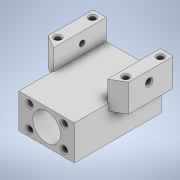
# Autodesk Inventor part: Губка-2
Saved by Autodesk Inventor 2022 (Build 260153000, 153)
## iProperties
Created: 2021-12-03
Part Number: Губка-2
Material: Типовые
Document SubType Name: Modeling
Designer: Украинцев
Density: 1 g/cm^3
Appearance: По умолчанию
Author: Украинцев
Autodesk Inventor part; units mm, degrees
ref_plane "YZ Plane" through (0, 0, 0) normal (1, 0, 0) x (0, 1, 0)
ref_plane "XZ Plane" through (0, 0, 0) normal (0, 1, 0) x (-1, 0, 0)
ref_plane "XY Plane" through (0, 0, 0) normal (0, 0, 1) x (1, 0, 0)
sketch "Эскиз1" plane through (0, 0, 0) normal (0, 1, 0) x (-1, 0, 0)
  line L0 (-40, 62.5) -> (40, 62.5)
  line L1 (40, 62.5) -> (40, -62.5)
  line L2 (40, -62.5) -> (-40, -62.5)
  line L3 (-40, -62.5) -> (-40, 62.5)
  line L4 (-40, 62.5) -> (40, -62.5) construction
  line L5 (40, 62.5) -> (-40, -62.5) construction
  line L6 (0, -62.5) -> (-58, -62.5)
  line L7 (-58, -62.5) -> (-58, 2.5)
  line L8 (-58, 2.5) -> (-39, 13.4697)
  line L9 (-58, -62.5) -> (-39, -62.5)
  line L10 (-39, -62.5) -> (-39, 13.4697)
  line L11 (0, 62.5) -> (0, -62.5)
  line L12 (0, -62.5) -> (58, -62.5)
  line L13 (58, -62.5) -> (58, 2.5)
  line L14 (58, 2.5) -> (39, 13.4697)
  line L15 (39, -62.5) -> (39, 13.4697)
  point P0 (0, 0)
  point P1 (-40, 12.8923)
  point P2 (40, 12.8923)
  dimension "d0" = 80
  dimension "d1" = 125
  dimension "d2" = 58
  dimension "d3" = 65
  dimension "d4" = 120
  dimension "d5" = 19
  constraints: 32 end point, 4 midpoint, 4 symmetric about line, 3 perpendicular, 2 horizontal, 2 parallel, 2 point on line, 1 vertical
  measures "d0" distance of L1.end L2.end
  measures "d1" distance of L0.end L1.end
  measures "d2" distance of L6.start L6.end
  measures "d3" distance of L6.end L7.end
  measures "d4" angle of L7 L8
  measures "d5" distance of L6.end L9.end
extrude "Выдавливание1" add sketch "Эскиз1" along normal blind 30 and the other way blind 10 contours L8 L10 L2 L3 | L3 L6 L7 L8 | L14 L13 L12 L1 | L1 L2 L15 L14
extrude "Выдавливание2" add sketch "Эскиз1" against normal blind 50 contours L0 L11 L2 L10 L8 L3 | L0 L1 L14 L15 L2 L11 | L8 L10 L2 L3 | L1 L2 L15 L14
sketch "Эскиз3" plane through (0, 30, 0) normal (0, 1, 0) x (1, 0, 0)
  line L0 (39, 62.5) -> (-39, 62.5) projected
  line L1 (0, 62.5) -> (49, 62.5)
  line L2 (49, 62.5) -> (49, 52.5)
  line L3 (49, 52.5) -> (49, 2.5)
  point P0 (0, 0)
  point P1 (40, 62.5)
  point P2 (-40, 62.5)
  dimension "d15" = 49
  dimension "d16" = 10
  dimension "d17" = 50
  constraints: 6 end point, 2 coincident, 1 collinear, 1 midpoint, 1 perpendicular, 1 point on line
  measures "d15" distance of L1.start L1.end
  measures "d16" distance of L1.end L2.end
  measures "d17" distance of L2.end L3.end
hole "Отверстие1" at (49, 30, -2.5) at (49, 30, -52.5) direction (0, -1, 0) diameter 8 depth 18 tip angle 118
thread "Резьба1" size "M8x1.25" class "6H" standard "ANSI Metric M Profile" length 13
thread "Резьба2" size "M8x1.25" class "6H" standard "ANSI Metric M Profile" length 13
sketch "Эскиз4" plane through (0, 30, 0) normal (0, 1, 0) x (1, 0, 0)
  line L0 (39, 62.5) -> (-39, 62.5) projected
  line L1 (0, 62.5) -> (-49, 62.5)
  line L2 (-49, 62.5) -> (-49, 52.5)
  line L3 (-49, 52.5) -> (-49, 2.5)
  point P0 (0, 0)
  dimension "d29" = 49
  dimension "d30" = 10
  dimension "d31" = 50
  constraints: 6 end point, 2 coincident, 1 collinear, 1 midpoint, 1 perpendicular, 1 point on line
  measures "d29" distance of L1.start L1.end
  measures "d30" distance of L1.end L2.end
  measures "d31" distance of L2.end L3.end
hole "Отверстие2" at (-49, 30, -52.5) at (-49, 30, -2.5) direction (0, -1, 0) diameter 8 depth 18 tip angle 118
thread "Резьба3" size "M8x1.25" class "6H" standard "ANSI Metric M Profile" length 13
thread "Резьба4" size "M8x1.25" class "6H" standard "ANSI Metric M Profile" length 13
sketch "Эскиз5" plane through (-40, 0, 62.5) normal (0, 0, 1) x (1, 0, 0)
  line L0 (40, 0) -> (40, -50)
  line L1 (0, -50) -> (80, -50) projected
  line L2 (0, -10) -> (0, -50) projected
  line L3 (0, -25) -> (80, -25)
  line L4 (80, -10) -> (80, -50) projected
  line L5 (15, -41) -> (65, -41)
  line L6 (65, -41) -> (65, -9)
  line L7 (65, -9) -> (15, -9)
  line L8 (15, -9) -> (15, -41)
  line L9 (15, -41) -> (65, -9) construction
  line L10 (65, -41) -> (15, -9) construction
  point P0 (40, -25)
  dimension "d44" = 50
  dimension "d45" = 32
  constraints: 16 end point, 4 coincident, 2 parallel, 2 perpendicular, 2 point on line, 1 horizontal, 1 midpoint
  measures "d44" distance of L7.end L6.end
  measures "d45" distance of L6.end L5.end
hole "Отверстие3" at (0, -25, 62.5) direction (0, 0, -1) diameter 40 end through all
hole "Отверстие4" at (25, -41, 62.5) at (-25, -41, 62.5) at (-25, -9, 62.5) at (25, -9, 62.5) direction (0, 0, -1) diameter 8 depth 18 tip angle 118
thread "Резьба5" size "M8x1.25" class "6H" standard "ANSI Metric M Profile" length 13
thread "Резьба6" size "M8x1.25" class "6H" standard "ANSI Metric M Profile" length 13
thread "Резьба7" size "M8x1.25" class "6H" standard "ANSI Metric M Profile" length 13
thread "Резьба8" size "M8x1.25" class "6H" standard "ANSI Metric M Profile" length 13
sketch "Эскиз6" plane through (58, -10, -62.5) normal (1, 0, 0) x (0, 0, -1)
  line L0 (0, 10) -> (0, 40) projected
  line L1 (0, 10) -> (0, 25)
  line L2 (0, 25) -> (-35, 25)
  point P0 (-62.5, 10)
  dimension "d69" = 15
  dimension "d70" = 35
  constraints: 4 end point, 1 coincident, 1 midpoint, 1 perpendicular
  measures "d69" distance of L0.start L1.end
  measures "d70" distance of L1.end L2.end
hole "Отверстие5" at (58, 15, -27.5) direction (-1, 0, 0) diameter 8 depth 116
chamfer "Фаска1" distance 1.6 angle 45 1 edges at (-58, 15, -23.5)
chamfer "Фаска2" distance 1.6 angle 45 1 edges at (58, 15, -23.5)
chamfer "Фаска3" distance 1.6 angle 45 4 edges at (-25, -37, 62.5) (25, -37, 62.5) (-25, -5, 62.5) (25, -5, 62.5)
thread "Резьба9" size "M8x1.25" class "6H" standard "ANSI Metric M Profile" full length
chamfer "Фаска4" distance 1.6 angle 45 4 edges at (49, 30, -56.5) (49, 30, -6.5) (-49, 30, -56.5) (-49, 30, -6.5)
chamfer "Фаска5" distance 2 angle 45 2 edges at (58, 10, -62.5) (-58, 10, -62.5)
